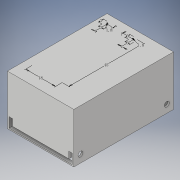
# Autodesk Inventor part: Case
Saved by Autodesk Inventor 2019 (Build 230136000, 136)
## iProperties
Created: 2019-12-10
Part Number: Case
Material: 常规
Document SubType Name: Modeling
Designer: cxcyh
Density: 1 g/cm^3
Appearance: 默认
Author: cxcyh
Autodesk Inventor part; units mm, degrees
ref_plane "YZ Plane" through (0, 0, 0) normal (1, 0, 0) x (0, 1, 0)
ref_plane "XZ Plane" through (0, 0, 0) normal (0, 1, 0) x (-1, 0, 0)
ref_plane "XY Plane" through (0, 0, 0) normal (0, 0, 1) x (1, 0, 0)
sketch "草图2" plane through (0, 0, 0) normal (0, 1, 0) x (-1, 0, 0)
  line L0 (-20, 30) -> (20, 30)
  line L1 (20, 30) -> (20, -30)
  line L2 (20, -30) -> (-20, -30)
  line L3 (-20, -30) -> (-20, 30)
  line L4 (-20, 30) -> (20, -30) construction
  line L5 (20, 30) -> (-20, -30) construction
  point P0 (0, 0)
  dimension "d15" = 40
  dimension "d16" = 60
  constraints: 12 end point, 2 midpoint, 2 parallel, 1 horizontal, 1 perpendicular
  measures "d15" distance of L1.end L2.end
  measures "d16" distance of L0.end L1.end
extrude "拉伸2" add sketch "草图2" along normal blind 30
shell "抽壳1" thickness 2 removed faces 1 at (-6.6667, 0, -10)
sketch "草图3" plane through (-20, 0, 30) normal (0, 0, 1) x (1, 0, 0)
  line L0 (40, 0) -> (0, 0) construction
  line L1 (40, 0) -> (40, 30) construction
  line L2 (0, 30) -> (40, 30) construction
  line L3 (0, 0) -> (0, 30) construction
  line L4 (0, 0) -> (0, 30) construction
  line L5 (40, 0) -> (40, 30) construction
  line L6 (40, 0) -> (0, 0) construction
  line L7 (3, 6.7398) -> (1, 6.7398)
  line L8 (1, 6.7398) -> (1, 0.7398)
  line L9 (0, 1.7398) -> (40, 1.7398) construction
  line L10 (3, 6.7398) -> (3, 2.7398)
  line L11 (40, 30) -> (0, 30) construction
  line L12 (20, 30) -> (20, 0) construction
  line L13 (38, 0) -> (2, 0) projected
  line L14 (3, 2.7398) -> (20, 2.7398)
  line L15 (1, 0.7398) -> (20, 0.7398)
  line L16 (37, 6.7398) -> (39, 6.7398)
  line L17 (39, 6.7398) -> (39, 0.7398)
  line L18 (37, 6.7398) -> (37, 2.7398)
  line L19 (37, 2.7398) -> (20, 2.7398)
  line L20 (39, 0.7398) -> (20, 0.7398)
  point P0 (20, 0)
  dimension "d29" = 2
  dimension "d44" = 5
  dimension "d45" = 2
  dimension "d46" = 6
  dimension "d47" = 40
  constraints: 24 end point, 5 point on line, 4 symmetric about line, 3 horizontal, 3 perpendicular, 2 midpoint
  measures "d29" distance from line of L7.start L8
  measures "d44" distance between parallel lines of L9 L7
  measures "d45" distance between parallel lines of L15 L14
  measures "d46" distance between parallel lines of L15 L7
  measures "d47" diameter of L1 L12
extrude "拉伸3" cut sketch "草图3" against normal blind 58
sketch "草图5" plane through (20, 0, 30) normal (1, 0, 0) x (0, 0, -1)
  line L0 (0, 6.7398) -> (58, 6.7398) construction
  line L1 (0, 0.7398) -> (58, 0.7398) construction
  line L2 (0, 6.7398) -> (2, 6.7398) construction
  line L3 (0, 2.7398) -> (2, 2.7398) construction
  line L4 (0, 2.7398) -> (58, 2.7398) construction
  line L5 (58, 6.7398) -> (2, 6.7398) construction
  line L6 (58, 6.7398) -> (58, 0.7398) construction
  line L7 (0, 0) -> (0, 30) construction
  line L8 (0, 4.7398) -> (58, 4.7398) construction
  circle A0 centre (4, 4.7398) radius 1.5
  line L9 (2, 0.7398) -> (2, 6.7398) construction
  circle A1 centre (56, 4.7398) radius 1.5
  point P0 (30, 0)
  dimension "d48" = 4
  dimension "d49" = 3
  dimension "d51" = 2
  dimension "d52" = 2
  dimension "d53" = 3
  dimension "d54" = 2
  constraints: 8 end point, 6 point on line, 3 perpendicular, 2 centre point, 1 horizontal
  measures "d48" diameter of L0 L8
  measures "d49" diameter of A0
  measures "d51" distance between parallel lines of L7 L9
  measures "d52" distance from line of A0.centre L9
  measures "d53" diameter of A1
  measures "d54" distance of L8.end A1.centre
extrude "拉伸4" cut sketch "草图5" against normal blind 2
mirror "镜像1" about plane through (0, 0, 0) normal (1, 0, 0) of "拉伸4"
sketch "草图7" plane through (-18, 28, 28) normal (0, -1, 0) x (1, 0, 0)
  line L0 (0, 0) -> (36, 0) construction
  line L1 (0, -56) -> (0, 0) construction
  line L2 (36, -56) -> (0, -56) construction
  line L3 (36, 0) -> (36, -56) construction
  line L4 (0.5, -55.5) -> (18.5, -55.5) construction
  line L5 (18.5, -55.5) -> (18.5, -10.5) construction
  line L6 (18.5, -10.5) -> (0.5, -10.5) construction
  line L7 (0.5, -10.5) -> (0.5, -55.5) construction
  circle A0 centre (17.5, -54.5) radius 0.9
  line L8 (19, -56) -> (16, -56)
  line L9 (16, -56) -> (16, -53)
  line L10 (16, -53) -> (19, -53)
  line L11 (19, -53) -> (19, -56)
  line L12 (19, -56) -> (16, -53) construction
  line L13 (16, -56) -> (19, -53) construction
  circle A1 centre (1.5, -54.5) radius 0.9
  line L14 (3, -56) -> (0, -56)
  line L15 (0, -56) -> (0, -53)
  line L16 (0, -53) -> (3, -53)
  line L17 (3, -53) -> (3, -56)
  line L18 (3, -56) -> (0, -53) construction
  line L19 (0, -56) -> (3, -53) construction
  line L20 (36, -56) -> (0, -56) projected
  line L21 (0, -56) -> (0, 0) projected
  dimension "d70" = 18
  dimension "d71" = 45
  dimension "d74" = 1.8
  dimension "d75" = 3
  dimension "d76" = 3
  dimension "d77" = 1
  dimension "d78" = 1
  dimension "d79" = 1.8
  dimension "d80" = 1
  dimension "d81" = 1
  dimension "d82" = 3
  dimension "d83" = 3
  constraints: 32 end point, 6 parallel, 4 midpoint, 3 horizontal, 3 perpendicular, 2 centre point, 2 collinear
  measures "d70" distance of L6.end L5.end
  measures "d71" distance of L5.end L4.end
  measures "d74" diameter of A0
  measures "d75" distance of L9.end L10.end
  measures "d76" distance of L8.end L9.end
  measures "d77" distance from line of L4 A0.centre
  measures "d78" distance from line of L5 A0.centre
  measures "d79" diameter of A1
  measures "d80" distance from line of L7 A1.centre
  measures "d81" distance from line of L4 A1.centre
  measures "d82" distance of L15.end L16.end
  measures "d83" distance of L14.end L15.end
